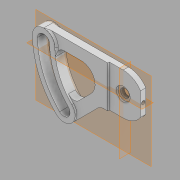
# Autodesk Inventor part: Pieza2A01209499
Saved by Autodesk Inventor 2020 (Build 240168000, 168)
## iProperties
Created: 2019-09-05
Part Number: Pieza2A01209499
Material: Genérico
Document SubType Name: Modeling
Designer: gerar
Density: 1 g/cm^3
Appearance: Valor por defecto
Author: gerar
Autodesk Inventor part; units mm, degrees
sketch "Boceto1" plane through (0, 0, 0) normal (0, 0, 1) x (1, 0, 0)
  line L0 (-37.2583, 0) -> (45.75, 0) construction
  line L1 (0, -58.9269) -> (0, 58.9269) construction
  line L2 (31.75, -21.0606) -> (31.75, 21.0606)
  line L3 (0, 38.1) -> (-25.4, 38.1)
  line L4 (0, -38.1) -> (-25.4, -38.1)
  arc A0 (31.75, 21.0606) -> (0, 38.1) centre (0, 0) ccw
  arc A1 (0, -38.1) -> (31.75, -21.0606) centre (0, 0) ccw
  line L5 (-25.4, 38.1) -> (-25.4, -38.1)
  dimension "d2" = 31.75
  dimension "d3" = 25.4
  constraints: 8 end point, 4 point on circle, 2 centre point, 2 horizontal, 2 tangent, 1 coincident, 1 parallel, 1 perpendicular, 1 vertical
  measures "d2" distance from line of L2 point (0, 0)
  measures "d3" distance of L3.end L3.start
extrude "Cabezal" add sketch "Boceto1" along normal blind 9.652
sketch "Boceto3" plane through (0, 0, 9.652) normal (0, 0, 1) x (1, 0, 0)
  point P0 (0, 0)
  point P1 (0, 0)
  constraints: 1 coincident
hole "Broca y barreno" at (0, 0, 9.652) direction (0, 0, -1) diameter 15.875 end through all counterbore diameter 25.4 counterbore depth 3.048
sketch "Boceto4" plane through (0, 0, 0) normal (0, 0, 1) x (1, 0, 0)
  line L0 (-36.83, 0) -> (43.18, 0) construction
  line L1 (0, -53.34) -> (0, 53.34) construction
  line L2 (-12.7, 17.526) -> (-227.4102, 17.526) construction
  arc A0 (-119.126, 17.526) -> (-160.274, 17.526) centre (-139.7, 17.526) ccw
  line L3 (-12.7, 17.526) -> (-138.4236, -108.1976) construction
  line L4 (-12.7, 17.526) -> (165.1, 17.526) construction
  arc A1 (-117.0506, -86.8246) -> (-87.9545, -57.7285) centre (-102.5026, -72.2766) ccw
  arc A2 (-160.274, 17.526) -> (-117.0506, -86.8246) centre (-12.7, 17.526) ccw
  arc A3 (-119.126, 17.526) -> (-87.9545, -57.7285) centre (-12.7, 17.526) ccw
  line L5 (-25.4, 38.1) -> (-25.4, -38.1) projected
  point P0 (0, 0)
  dimension "d14" = 17.526
  dimension "d15" = 12.7
  dimension "d19" = 41.148
  dimension "d21" = 135
  dimension "d22" = 41.148
  dimension "d25" = 12.7
  constraints: 8 point on circle, 6 end point, 5 point on line, 4 centre point, 2 coincident, 2 horizontal, 1 equal length
  measures "d14" vertical distance of point (0, 0) L2.start
  measures "d15" horizontal distance of point (0, 0) L2.start
  measures "d19" diameter of A0
  measures "d21" angle of L3 L4
  measures "d22" diameter of A1
  measures "d25" horizontal distance of L2.start L5.start
extrude "Mango" add sketch "Boceto4" along normal blind 15.875 and the other way blind 3.175
sketch "Boceto8" plane through (31.75, -21.0606, 0) normal (1, 0, 0) x (0, 0, -1)
  circle A0 centre (-4.826, 21.0606) radius 3.175
  line L0 (-9.652, 0) -> (-9.652, 42.1211) construction
  line L1 (0, 0) -> (-9.652, 0) construction
  line L2 (0, 42.1211) -> (-9.652, 42.1211) construction
  line L3 (-6.604, 33.7606) -> (-6.604, 8.3606) projected
  line L4 (-6.604, 28.9981) -> (-6.604, 13.1231) projected
  point P0 (0, 21.0606)
  dimension "d36" = 6.35
  dimension "d37" = 4.826
  dimension "d38" = 42.1211
  dimension "d39" = 21.0606
  constraints: 1 centre point, 1 coincident
  measures "d36" diameter of A0
  measures "d37" distance from line of L0 A0.centre
  measures "d38" distance between parallel lines of L1 L2
  measures "d39" distance from line of L2 A0.centre
extrude "AgujeroLateral" cut sketch "Boceto8" against normal blind 9.652
sketch "Boceto9" plane through (0, 0, 0) normal (0, 0, 1) x (1, 0, 0)
  arc A0 (-160.274, 17.526) -> (-119.126, 17.526) centre (-139.7, 17.526) ccw projected
  line L0 (-25.4, 38.1) -> (-25.4, -38.1) projected
  line L1 (-139.7, 38.1) -> (-25.4, 38.1)
  arc A1 (-119.126, 17.526) -> (-160.274, 17.526) centre (-139.7, 17.526) ccw projected
  line L2 (-25.4, -38.1) -> (0, -38.1) projected
  line L3 (-25.4, 38.1) -> (-25.4, -38.1)
  line L4 (-25.4, -38.1) -> (-33.9695, -38.1)
  arc A2 (-87.9545, -57.7285) -> (-117.0506, -86.8246) centre (-102.5026, -72.2766) ccw projected
  arc A3 (-160.274, 17.526) -> (-117.0506, -86.8246) centre (-12.7, 17.526) ccw projected
  arc A4 (-117.0506, -86.8246) -> (-87.9545, -57.7285) centre (-102.5026, -72.2766) ccw projected
  arc A5 (-119.126, 17.526) -> (-87.9545, -57.7285) centre (-12.7, 17.526) ccw projected
  arc A6 (-119.126, 17.526) -> (-160.274, 17.526) centre (-139.7, 17.526) ccw projected
  line L5 (10.5292, 11.6592) -> (185.2985, 11.6592) construction
  arc A7 (-117.0506, -86.8246) -> (-87.9545, -57.7285) centre (-102.5026, -72.2766) ccw construction
  line L6 (-87.9545, -86.8246) -> (-42.9497, -41.8197)
  line L7 (-139.7, 17.526) -> (0, 17.526) construction
  line L8 (0, 17.526) -> (-119.126, -101.6) construction
  arc A8 (-33.9695, -38.1) -> (-42.9497, -41.8197) centre (-33.9695, -50.8) ccw
  line L9 (-25.4, 38.1) -> (-25.4, -38.1)
  arc A9 (-87.9545, -57.7285) -> (-119.126, 17.526) centre (-12.7, 17.526) ccw projected
  arc A10 (-119.126, 17.526) -> (-87.9545, -57.7285) centre (-12.7, 17.526) ccw
  circle A11 centre (-139.7, 17.526) radius 20.574
  circle A12 centre (-102.5026, -72.2766) radius 20.574
  point P0 (0, 0)
  point P1 (-87.9545, -57.7285)
  point P2 (-119.126, 17.526)
  dimension "d47" = 45
  dimension "d48" = 12.7
  constraints: 16 end point, 6 point on circle, 5 tangent, 4 centre point, 3 perpendicular, 2 coincident, 2 concentric, 2 horizontal, 1 vertical
  measures "d47" angle of L7 L8
  measures "d48" radius of A8
extrude "BloqueCentral" add sketch "Boceto9" along normal blind 12.7 contours A9 L1 L0 L4 A8 L6 A5 | A1 L1 A9 | A9 L6 A4
sketch "Boceto10" plane through (0, 0, 15.875) normal (0, 0, 1) x (1, 0, 0)
  arc A0 (-160.274, 17.526) -> (-117.0506, -86.8246) centre (-12.7, 17.526) ccw construction
  arc A1 (-117.0506, -86.8246) -> (-87.9545, -57.7285) centre (-102.5026, -72.2766) ccw construction
  arc A2 (-119.126, 17.526) -> (-87.9545, -57.7285) centre (-12.7, 17.526) ccw construction
  arc A3 (-119.126, 17.526) -> (-160.274, 17.526) centre (-139.7, 17.526) ccw construction
  arc A4 (-150.876, 17.526) -> (-110.4052, -80.1792) centre (-12.7, 17.526) ccw
  arc A5 (-110.4052, -80.1792) -> (-94.5999, -64.3739) centre (-102.5026, -72.2766) ccw
  arc A6 (-128.524, 17.526) -> (-94.5999, -64.3739) centre (-12.7, 17.526) ccw
  arc A7 (-128.524, 17.526) -> (-150.876, 17.526) centre (-139.7, 17.526) ccw
  point P0 (0, 0)
  dimension "d52" = 22.352
  constraints: 8 point on circle, 4 centre point, 3 other
  measures "d52" radial gap between concentric circles of A6 A4
extrude "HuecoMango" cut sketch "Boceto10" against normal blind 22.352
sketch "Boceto11" plane through (0, 0, 12.7) normal (0, 0, 1) x (1, 0, 0)
  arc A0 (-105.5616, 17.526) -> (-118.1445, 3.1051) centre (-105.5616, 4.826) ccw
  arc A1 (-97.4576, -46.8374) -> (-78.3631, -48.1371) centre (-87.3433, -39.1568) ccw
  arc A2 (-56.0605, -25.8345) -> (-74.021, 17.526) centre (-74.021, -7.874) ccw
  arc A3 (-128.524, 17.526) -> (-150.876, 17.526) centre (-139.7, 17.526) ccw construction
  arc A4 (-128.524, 17.526) -> (-94.5999, -64.3739) centre (-12.7, 17.526) ccw construction
  arc A5 (-110.4052, -80.1792) -> (-94.5999, -64.3739) centre (-102.5026, -72.2766) ccw construction
  arc A6 (-150.876, 17.526) -> (-110.4052, -80.1792) centre (-12.7, 17.526) ccw construction
  arc A7 (-119.126, 17.526) -> (-160.274, 17.526) centre (-139.7, 17.526) ccw construction
  arc A8 (-160.274, 17.526) -> (-117.0506, -86.8246) centre (-12.7, 17.526) ccw construction
  arc A9 (-117.0506, -86.8246) -> (-87.9545, -57.7285) centre (-102.5026, -72.2766) ccw construction
  arc A10 (-119.126, 17.526) -> (-87.9545, -57.7285) centre (-12.7, 17.526) ccw construction
  line L0 (-139.7, 17.526) -> (-12.7, 17.526) construction
  line L1 (-12.7, 17.526) -> (-102.5026, -72.2766) construction
  arc A11 (-119.126, 17.526) -> (-87.9545, -57.7285) centre (-12.7, 17.526) ccw projected
  line L2 (-150.876, 17.526) -> (-150.876, 17.526)
  line L3 (-110.0905, -79.8645) -> (-110.4052, -80.1792)
  line L4 (-78.3631, -48.1371) -> (-56.0605, -25.8345)
  line L5 (-105.5616, 17.526) -> (-74.021, 17.526)
  arc A12 (-118.1445, 3.1051) -> (-97.4576, -46.8374) centre (-12.7, 17.526) ccw
  line L6 (-87.9545, -86.8246) -> (-42.9497, -41.8197) projected
  line L7 (-25.4, 38.1) -> (-139.7, 38.1) projected
  point P0 (0, 0)
  dimension "d57" = 25.4
  dimension "d58" = 25.4
  dimension "d59" = 50.8
  dimension "d60" = 20.574
  dimension "d61" = 20.574
  constraints: 13 point on circle, 12 end point, 10 tangent, 4 centre point, 3 horizontal, 2 collinear
  measures "d57" diameter of A0
  measures "d58" diameter of A1
  measures "d59" diameter of A2
  measures "d60" distance between parallel lines of L6 L4
  measures "d61" distance between parallel lines of L5 L7
extrude "HuecoCentral" cut sketch "Boceto11" against normal blind 12.7
fillet "Empalme1" radius 3.048 4 edges at (-118.8803, 10.2989, 12.7) (-125.152, 32.074, 12.7) (-118.8803, 10.2989, 0) (-125.152, 32.074, 0)
equation "\"d39\" = 0.5 * d38"
